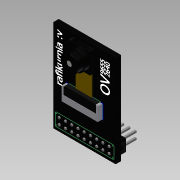
# Autodesk Inventor part: ov9655
Saved by Autodesk Inventor 2015 SP1 (Build 190203100, 203)
## iProperties
Created: 2015-02-02
Part Number: ov9655
Material: Generic
Document SubType Name: Modeling
Designer: Rafi Kurnia Putra
Density: 1 g/cm^3
Appearance: Default
Mass: 2.67153 g
Surface Area: 26.9729 cm^2
Volume: 2.67153 cm^3
Author: Rafi Kurnia Putra
Autodesk Inventor part; units mm, degrees
ref_plane "YZ Plane" through (0, 0, 0) normal (1, 0, 0) x (0, 1, 0)
ref_plane "XZ Plane" through (0, 0, 0) normal (0, 1, 0) x (-1, 0, 0)
ref_plane "XY Plane" through (0, 0, 0) normal (0, 0, 1) x (1, 0, 0)
sketch "Sketch1" plane through (0, 0, 0) normal (0, 1, 0) x (-1, 0, 0)
  line L0 (12.16, -17.95) -> (-12.16, -17.95)
  line L1 (-12.16, -17.95) -> (-12.16, 17.95)
  line L2 (-12.16, 17.95) -> (12.16, 17.95)
  line L3 (12.16, 17.95) -> (12.16, -17.95)
  line L4 (12.16, -17.95) -> (-12.16, 17.95) construction
  line L5 (-12.16, -17.95) -> (12.16, 17.95) construction
  line L6 (4.11, -16.95) -> (-4.11, -16.95)
  line L7 (-4.11, -16.95) -> (-4.11, -8.9)
  line L8 (-4.11, -8.9) -> (4.11, -8.9)
  line L9 (4.11, -8.9) -> (4.11, -16.95)
  line L10 (4.11, -16.95) -> (-4.11, -8.9) construction
  line L11 (-4.11, -16.95) -> (4.11, -8.9) construction
  circle A0 centre (0, -12.925) radius 3.94
  circle A1 centre (0, -12.925) radius 3.42
  line L12 (3.025, -0.27) -> (-3.025, -0.27)
  line L13 (-3.025, -0.27) -> (-3.025, -8.9)
  line L14 (-3.025, -8.9) -> (3.025, -8.9)
  line L15 (3.025, -8.9) -> (3.025, -0.27)
  line L16 (3.025, -0.27) -> (-3.025, -8.9) construction
  line L17 (-3.025, -0.27) -> (3.025, -8.9) construction
  line L18 (6.06, -0.27) -> (6.06, -0.02)
  line L19 (6.06, -0.02) -> (7.06, -0.02)
  line L20 (-6.06, -0.27) -> (-6.06, -0.02)
  line L21 (-6.06, -0.02) -> (-7.06, -0.02)
  line L22 (7.06, -0.02) -> (7.06, 5.31)
  line L23 (7.06, 5.31) -> (-7.06, 5.31)
  line L24 (-7.06, 5.31) -> (-7.06, -0.02)
  circle A2 centre (9.728, 15.518) radius 0.5
  circle A3 centre (7.296, 15.518) radius 0.5
  circle A4 centre (4.864, 15.518) radius 0.5
  circle A5 centre (2.432, 15.518) radius 0.5
  circle A6 centre (0, 15.518) radius 0.5
  circle A7 centre (-2.432, 15.518) radius 0.5
  circle A8 centre (-4.864, 15.518) radius 0.5
  circle A9 centre (-7.296, 15.518) radius 0.5
  circle A10 centre (-9.728, 15.518) radius 0.5
  circle A11 centre (9.728, 13.086) radius 0.5
  circle A12 centre (7.296, 13.086) radius 0.5
  circle A13 centre (4.864, 13.086) radius 0.5
  circle A14 centre (2.432, 13.086) radius 0.5
  circle A15 centre (0, 13.086) radius 0.5
  circle A16 centre (-2.432, 13.086) radius 0.5
  circle A17 centre (-4.864, 13.086) radius 0.5
  circle A18 centre (-7.296, 13.086) radius 0.5
  circle A19 centre (-9.728, 13.086) radius 0.5
  line L25 (0, 13.086) -> (0, 15.518)
  line L26 (11.48, 16.792) -> (-11.48, 16.792)
  line L27 (-11.48, 16.792) -> (-11.48, 11.812)
  line L28 (-11.48, 11.812) -> (11.48, 11.812)
  line L29 (11.48, 11.812) -> (11.48, 16.792)
  line L30 (11.48, 16.792) -> (-11.48, 11.812) construction
  line L31 (-11.48, 16.792) -> (11.48, 11.812) construction
  line L32 (-6.06, -0.27) -> (-3.025, -0.27)
  line L33 (3.025, -0.27) -> (6.06, -0.27)
  point P0 (0, 0)
  point P1 (0, -4.585)
  point P2 (0, -8.9)
  point P3 (0, 14.302)
  dimension "d0" = 24.32
  dimension "d1" = 35.9
  dimension "d2" = 8.22
  dimension "d3" = 8.05
  dimension "d4" = 1
  dimension "d5" = 8.05
  dimension "d6" = 8.05
  dimension "d7" = 7.88
  dimension "d8" = 6.84
  dimension "d9" = 6.05
  dimension "d10" = 8.63
  dimension "d13" = 0.25
  dimension "d14" = 1
  dimension "d15" = 90
  dimension "d16" = 0.25
  dimension "d17" = 1
  dimension "d18" = 90
  dimension "d19" = 5.33
  dimension "d21" = 2.432
  dimension "d22" = 2.432
  dimension "d23" = 1
  dimension "d26" = 2.432
  dimension "d29" = 2.432
  dimension "d32" = 22.96
  dimension "d33" = 4.98
  constraints: 68 end point, 20 centre point, 11 midpoint, 9 perpendicular, 8 parallel, 6 horizontal, 5 vertical, 2 coincident, 34 other
  measures "d0" distance of L1.end L2.end
  measures "d1" distance of L0.end L1.end
  measures "d2" distance of L7.end L8.end
  measures "d3" distance of L6.end L7.end
  measures "d4" distance between parallel lines of L6 L0
  measures "d5" distance between parallel lines of L9 L3
  measures "d6" distance between parallel lines of L1 L7
  measures "d7" diameter of A0
  measures "d8" diameter of A1
  measures "d9" distance of L14.end L13.end
  measures "d10" distance of L13.end L12.end
  measures "d13" distance of L18.start L18.end
  measures "d14" distance of L18.end L19.end
  measures "d15" angle of L18 L19
  measures "d16" distance of L20.start L20.end
  measures "d17" distance of L20.end L21.end
  measures "d18" angle of L21 L20
  measures "d19" distance of L19.end L22.end
  measures "d21" distance from line of L2 A2.centre
  measures "d22" distance from line of L3 A2.centre
  measures "d23" diameter of A2
  measures "d26" distance of A2.centre A3.centre
  measures "d29" distance of A2.centre A11.centre
  measures "d32" distance of L28.end L27.end
  measures "d33" distance of L27.end L26.end
extrude "Extrusion1" add sketch "Sketch1" along normal blind 2.09 contours L0 L1 L2 L3 | L12 L32 L20 L21 L24 L23 L22 L19 L18 L33
extrude "Extrusion2" add sketch "Sketch1" along normal blind 4.05 contours L6 L7 L8 L9
extrude "Extrusion3" add sketch "Sketch1" along normal blind 5.81 contours A0
extrude "Extrusion4" add sketch "Sketch1" along normal blind 8.1 contours A1
extrude "Extrusion5" add sketch "Sketch1" along normal blind 2.5 contours L8 L13 L12 L15
extrude "Extrusion6" add sketch "Sketch1" along normal blind 3.88 contours L12 L32 L20 L21 L24 L23 L22 L19 L18 L33
extrude "Extrusion7" add sketch "Sketch1" along normal blind 2.09 contours L29 L28 L27 L26
extrude "Extrusion8" add sketch "Sketch1" against normal blind 2.62 contours L29 L28 L27 L26
extrude "Extrusion9" add sketch "Sketch1" against normal blind 8.2 contours A2 | A3 | A4 | A5 | A6 | A7 | A8 | A9 | A10 | A11 | A12 | A13 | A14 | A15 | A16 | A17 | A18 | A19
extrude "Extrusion10" add sketch "Sketch1" along normal blind 2.5 contours A2 | A3 | A4 | A5 | A6 | A7 | A8 | A9 | A10 | A11 | A12 | A13 | A14 | A15 | A16 | A17 | A18 | A19
fillet "Fillet1" radius 0.25 36 edges at (10.228, -8.2, 15.518) (10.228, -8.2, 13.086) (7.796, -8.2, 15.518) (7.796, -8.2, 13.086) (5.364, -8.2, 15.518) (5.364, -8.2, 13.086) (2.932, -8.2, 15.518) (2.932, -8.2, 13.086) (0.5, -8.2, 15.518) (0.5, -8.2, 13.086) (-1.932, -8.2, 15.518) (-1.932, -8.2, 13.086) (-4.364, -8.2, 15.518) (-4.364, -8.2, 13.086) (-6.796, -8.2, 15.518) (-6.796, -8.2, 13.086) (-9.228, -8.2, 15.518) (-9.228, -8.2, 13.086) (10.228, 2.5, 15.518) (10.228, 2.5, 13.086) (7.796, 2.5, 15.518) (7.796, 2.5, 13.086) (5.364, 2.5, 15.518) (5.364, 2.5, 13.086) (2.932, 2.5, 15.518) (2.932, 2.5, 13.086) (0.5, 2.5, 15.518) (0.5, 2.5, 13.086) (-1.932, 2.5, 15.518) (-1.932, 2.5, 13.086) (-4.364, 2.5, 13.086) (-4.364, 2.5, 15.518) (-6.796, 2.5, 15.518) (-6.796, 2.5, 13.086) (-9.228, 2.5, 13.086) (-9.228, 2.5, 15.518)
fillet "Fillet2" radius 0.5 4 edges at (11.48, -1.31, 16.792) (11.48, -1.31, 11.812) (-11.48, -1.31, 11.812) (-11.48, -1.31, 16.792)
fillet "Fillet3" radius 0.125 10 edges at (4.11, 4.05, -12.925) (4.11, 3.07, -16.95) (0, 4.05, -16.95) (-4.11, 3.07, -16.95) (4.11, 3.07, -8.9) (0, 4.05, -8.9) (-4.11, 3.07, -8.9) (-4.11, 4.05, -12.925) (3.94, 5.81, -12.925) (3.42, 8.1, -12.925)
sketch "Sketch2" plane through (0, 3.88, 0) normal (0, 1, 0) x (1, 0, 0)
  line L0 (-7.06, 0.02) -> (-7.06, -5.31)
  line L1 (-7.06, -5.31) -> (7.06, -5.31)
  line L2 (7.06, -5.31) -> (7.06, 0.02)
  line L3 (-6.36, -2.9) -> (6.36, -2.9)
  line L4 (6.36, -2.9) -> (6.36, 0.02)
  line L5 (-6.36, 0.02) -> (-6.36, -2.9)
  line L6 (6.36, 0.02) -> (7.06, 0.02)
  line L7 (-7.06, 0.02) -> (-6.36, 0.02)
  point P0 (0, 0)
  dimension "d60" = 0.7
  dimension "d61" = 0.7
  dimension "d62" = 2.41
  constraints: 16 end point, 3 vertical, 2 horizontal, 1 perpendicular
  measures "d60" distance from line of L5.start L0
  measures "d61" distance between parallel lines of L4 L2
  measures "d62" distance between parallel lines of L3 L1
extrude "Extrusion11" add sketch "Sketch2" along normal blind 0.1
sketch "Sketch3" plane through (0, 8.1, -12.925) normal (0, 1, 0) x (1, 0, 0)
  circle A0 centre (0, 0) radius 1
  point P0 (0, -12.925)
  dimension "d65" = 2
  constraints: 1 centre point
  measures "d65" diameter of A0
extrude "Extrusion12" cut sketch "Sketch3" against normal blind 0.1
sketch "Sketch4" plane through (0, 2.09, 0) normal (0, 1, 0) x (1, 0, 0)
  line L0 (6.1843, 3.5352) -> (6.1843, 9.8545) construction
  line L1 (6.1843, 9.8545) -> (9.8318, 9.8545) construction
  line L2 (9.8318, 9.8545) -> (9.8318, 3.5352) construction
  line L3 (9.8318, 3.5352) -> (6.1843, 3.5352) construction
  line L4 (6.1836, 10.0499) -> (6.1836, 17.674) construction
  line L5 (6.1836, 17.674) -> (8.7453, 17.674) construction
  line L6 (8.7453, 17.674) -> (8.7453, 10.0499) construction
  line L7 (8.7453, 10.0499) -> (6.1836, 10.0499) construction
  line L8 (8.1541, 10.0472) -> (8.1541, 17.6713) construction
  line L9 (8.1541, 17.6713) -> (10.7158, 17.6713) construction
  line L10 (10.7158, 17.6713) -> (10.7158, 10.0472) construction
  line L11 (10.7158, 10.0472) -> (8.1541, 10.0472) construction
  line L12 (-10.98, -16.792) -> (10.98, -16.792) projected
  line L13 (10.98, -11.812) -> (-10.98, -11.812) projected
  line L14 (-11.48, -12.312) -> (-11.48, -16.292) projected
  arc A0 (-11.48, -16.292) -> (-10.98, -16.792) centre (-10.98, -16.292) ccw projected
  arc A1 (-10.98, -11.812) -> (-11.48, -12.312) centre (-10.98, -12.312) ccw projected
  arc A2 (10.98, -16.792) -> (11.48, -16.292) centre (10.98, -16.292) ccw projected
  line L15 (11.48, -16.292) -> (11.48, -12.312) projected
  arc A3 (11.48, -12.312) -> (10.98, -11.812) centre (10.98, -12.312) ccw projected
  line L16 (-7.06, 0.02) -> (-7.06, -5.31) projected
  line L17 (-7.06, -5.31) -> (7.06, -5.31) projected
  line L18 (7.06, -5.31) -> (7.06, 0.02) projected
  line L19 (-7.06, 0.02) -> (-7.06, -5.31) projected
  line L20 (-7.06, -5.31) -> (7.06, -5.31) projected
  line L21 (7.06, -5.31) -> (7.06, 0.02) projected
  line L22 (7.06, 0.02) -> (6.36, 0.02) projected
  line L23 (6.36, 0.02) -> (6.36, -2.9) projected
  line L24 (6.36, -2.9) -> (-6.36, -2.9) projected
  line L25 (-6.36, -2.9) -> (-6.36, 0.02) projected
  line L26 (-6.36, 0.02) -> (-7.06, 0.02) projected
  line L27 (-6.36, 0.02) -> (-7.06, 0.02) projected
  line L28 (-6.06, 0.02) -> (-6.36, 0.02) projected
  line L29 (-6.06, 0.27) -> (-6.06, 0.02) projected
  line L30 (6.06, 0.27) -> (-6.06, 0.27) projected
  line L31 (7.06, 0.02) -> (6.36, 0.02) projected
  line L32 (6.36, 0.02) -> (6.06, 0.02) projected
  line L33 (6.06, 0.02) -> (6.06, 0.27) projected
  line L34 (6.36, 0.12) -> (7.16, 0.12)
  line L35 (7.16, 0.12) -> (7.16, -5.41)
  line L36 (7.16, -5.41) -> (-7.16, -5.41)
  line L37 (-7.16, -5.41) -> (-7.16, 0.12)
  line L38 (-7.16, 0.12) -> (-6.36, 0.12)
  circle A4 centre (0, 12.925) radius 1 projected
  circle A5 centre (0, 12.925) radius 1 projected
  circle A6 centre (0, 12.925) radius 3.295 projected
  circle A7 centre (0, 12.925) radius 1 projected
  point P0 (0, 0)
  dimension "d68" = 0.1
  constraints: 10 end point, 10 other
  measures "d68" distance between parallel lines of L17 L36
sketch "Sketch5" plane through (0, 8.1, -12.925) normal (0, 1, 0) x (1, 0, 0)
  circle A0 centre (0, 0) radius 1 projected
  circle A1 centre (0, 0) radius 3.295 projected
  line L0 (12.16, 5.025) -> (-12.16, 5.025) projected
  point P0 (0, -12.925)
sketch "Sketch6" plane through (0, 2.09, 0) normal (0, 1, 0) x (1, 0, 0)
  line L0 (-11.8218, -2.1963) -> (-11.8218, 23.4268) construction
  line L1 (-11.8218, 23.4268) -> (-8.0694, 23.4268) construction
  line L2 (-8.0694, 23.4268) -> (-8.0694, -2.1963) construction
  line L3 (-8.0694, -2.1963) -> (-11.8218, -2.1963) construction
  point P0 (0, 0)
  constraints: 2 other
body "Solid1"
